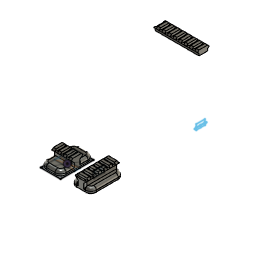
PhotoPicaTinny v1 (Autodesk Fusion 360 design; units mm, degrees)
Autodesk Fusion 360 part; units mm, degrees
sketch "Sketch1" plane through (0, 0, 0) normal (0, 0, 1) x (1, 0, 0)
  line L0 (18, 30) -> (-18, 30)
  line L1 (-18, 30) -> (-18, -30)
  line L2 (-18, -30) -> (18, -30)
  line L3 (18, -30) -> (18, 30)
  line L4 (18, 30) -> (-18, -30) construction
  line L5 (-18, 30) -> (18, -30) construction
  dimension "d1" = 36
  dimension "d2" = 60
  constraint horizontal L0
  constraint perpendicular L0 L1
  constraint parallel L0 L2
  constraint parallel L1 L3
  constraint coincident L4 origin
  constraint coincident L5 origin
  measures "d1" distance of L1.end L2.end
  measures "d2" distance of L0.end L1.end
extrude "Extrude1" add sketch "Sketch1" along normal blind 10 makes body 1
sketch "Sketch2" plane through (0, 0, 0) normal (0, 0, 1) x (1, 0, 0)
  line L0 (5, 30) -> (-5, 30)
  line L1 (-5, 30) -> (-5, -30)
  line L2 (-5, -30) -> (5, -30)
  line L3 (5, -30) -> (5, 30)
  line L4 (5, 30) -> (-5, -30) construction
  line L5 (-5, 30) -> (5, -30) construction
  line L6 (18, 30) -> (-18, 30)
  dimension "d5" = 10
  constraint horizontal L0
  constraint perpendicular L0 L1
  constraint parallel L0 L2
  constraint parallel L1 L3
  constraint coincident L4 origin
  constraint coincident L5 origin
  constraint coincident L0.start L6
  measures "d5" distance of L1.end L2.end
copy_body "CopyPasteBodies3" bodies 1 makes body 2
move_body "Move8" bodies 2 to x (1, 0, 0) y (0, 1, 0) z (0, 0, 1) at (0, 0, 0)
extrude "Extrude2" add sketch "Sketch2" along normal blind 13 bodies 1
sketch "Sketch3" plane through (0, 0, 0) normal (0, 0, 1) x (1, 0, 0)
sketch "Sketch4" plane through (0, 0, 0) normal (0, 0, 1) x (1, 0, 0)
  line L0 (18, 5) -> (-18, 5)
  line L1 (-18, 5) -> (-18, -5)
  line L2 (-18, -5) -> (18, -5)
  line L3 (18, -5) -> (18, 5)
  line L4 (18, 5) -> (-18, -5) construction
  line L5 (-18, 5) -> (18, -5) construction
  dimension "d8" = 10
  constraint horizontal L0
  constraint perpendicular L0 L1
  constraint parallel L0 L2
  constraint parallel L1 L3
  constraint coincident L4 origin
  constraint coincident L5 origin
  measures "d8" distance of L0.end L1.end
extrude "Extrude3" add sketch "Sketch1" along normal blind 10 separate body makes body 3
extrude "Extrude4" add sketch "Sketch4" along normal blind 12 separate body makes body 4
sketch "PicaMeasure2D" plane through (0, 0, 0) normal (1, 0, 0) x (0, 1, 0)
  line L0 (250.67, -64.32) -> (235, -64.32)
  line L1 (235, -64.32) -> (235, -55)
  line L2 (242.835, -61.32) -> (253.435, -61.32)
  line L3 (242.835, -61.32) -> (232.235, -61.32)
  line L4 (232.235, -61.32) -> (235, -64.32)
  line L5 (232.235, -61.32) -> (235, -58.7716)
  line L6 (249.8865, -60.32) -> (249.8865, -61.32)
  line L7 (242.835, -64.32) -> (242.835, -61.32)
  line L8 (242.835, -60.32) -> (249.8865, -60.32)
  line L9 (235, -55) -> (250.67, -55)
  line L10 (250.67, -55) -> (250.67, -64.32)
  line L11 (242.835, -61.32) -> (242.835, -60.32)
  line L12 (253.435, -61.32) -> (250.67, -58.7716)
  line L13 (242.835, -60.32) -> (235.7835, -60.32)
  line L14 (235.7835, -60.32) -> (235.7835, -61.32)
  line L15 (250.67, -64.32) -> (253.435, -61.32)
extrude "Extrude5" add sketch "PicaMeasure2D" along normal blind 5 separate body contours L2 L10 L12 | L1 L2 L3 L6 L8 L9 L10 L13 L14 | L1 L3 L5 makes body 5
extrude "Extrude6" add sketch "PicaMeasure2D" against normal blind 5 bodies 5
combine "Combine2" operation add target body 3 tool bodies 4
combine "Combine3" operation add target body 1 tool bodies 2
pattern_linear "R-Pattern1" count 8 spacing 10 along (1, 0, 0) of bodies 5 makes body 6 at (5, 240.2233, -60.6211) makes body 7 at (15, 240.2233, -60.6211) makes body 8 at (25, 240.2233, -60.6211) makes body 9 at (35, 240.2233, -60.6211) makes body 10 at (45, 240.2233, -60.6211) makes body 11 at (55, 240.2233, -60.6211) makes body 12 at (65, 240.2233, -60.6211)
combine "Combine1" operation add target body 5 tool bodies 6 7 8 9 10 11 12
move_body "Move1" bodies 5 to x (-1, 0, 0) y (0, 1, 0) z (0, 0, -1) at (0, 0, 0)
copy_body "CopyPasteBodies1" bodies 5 makes body 13
move_body "Move2" bodies 13 to x (1, 0, 0) y (0, 1, 0) z (0, 0, 1) at (57, -242.835, -43)
copy_body "CopyPasteBodies2" bodies 13 makes body 14
move_body "Move3" bodies 14 to x (0, 1, 0) y (-1, 0, 0) z (0, 0, 1) at (-25.835, 10.165, 0)
move_body "Move4" bodies 14 to x (1, 0, 0) y (0, 1, 0) z (0, 0, 1) at (25.835, -22.165, 1)
move_body "Move6" bodies 14 to x (1, 0, 0) y (0, 1, 0) z (0, 0, 1) at (0, -2, 0)
move_body "Move7" bodies 13 to x (1, 0, 0) y (0, 1, 0) z (0, 0, 1) at (-4, 0, 0)
sketch "Sketch6" plane through (58, 0, 0) normal (1, 0, 0) x (0, 1, 0)
  line L0 (-7.835, 21.32) -> (-10.6, 18.32)
  line L1 (-10.6, 18.32) -> (-7.835, 15.7716)
  line L2 (-7.835, 15.7716) -> (-7.835, 12)
  line L3 (-7.835, 12) -> (7.835, 12)
  line L4 (7.835, 12) -> (7.835, 15.7716)
  line L5 (7.835, 15.7716) -> (10.6, 18.32)
  line L6 (10.6, 18.32) -> (7.835, 21.32)
  line L7 (7.835, 21.32) -> (-7.835, 21.32)
  line L8 (8.4924, 22.82) -> (-8.4924, 22.82)
  line L9 (-8.4924, 22.82) -> (-12.7196, 18.2336)
  line L10 (-12.7196, 18.2336) -> (-9.335, 15.1142)
  line L11 (-9.335, 15.1142) -> (-9.335, 10.5)
  line L12 (-9.335, 10.5) -> (9.335, 10.5)
  line L13 (9.335, 10.5) -> (9.335, 15.1142)
  line L14 (9.335, 15.1142) -> (12.7196, 18.2336)
  line L15 (12.7196, 18.2336) -> (8.4924, 22.82)
  dimension "d48" = 1.5
extrude "Extrude8" add 1 faces at (-6, -5, 10.6667) along direction (0, -1, 0) blind 2.835 on bodies 3 bodies 3 13
extrude "Extrude10" cut sketch "Sketch1" along normal blind 30 keep common part bodies 3
extrude "Extrude11" add 1 faces at (-5, 10, 11) along direction (-1, 0, 0) blind 2.835 on bodies 1 bodies 1 14
extrude "Extrude12" add 1 faces at (5, -10, 11) along direction (1, 0, 0) blind 2.835 on bodies 1 bodies 1
extrude "Extrude13" cut sketch "Sketch1" along normal blind 25 keep common part bodies 1
move_body "Move5" bodies 1 to x (1, 0, 0) y (0, 1, 0) z (0, 0, 1) at (55, 0, 0)
extrude "Extrude15" add 1 faces at (6, 5, 10.6667) along direction (0, 1, 0) blind 2.835 on bodies 3 bodies 3
fillet "Fillet1" radius 10 8 edges at (37, -30, 5) (73, -30, 5) (73, 30, 5) (37, 30, 5) (18, -30, 5) (-18, -30, 5) (18, 30, 5) (-18, 30, 5) on bodies 1 3
fillet "Fillet2" radius 5 20 edges at (47.0825, 30, 10) (39.9289, 27.0711, 10) (37, 0, 10) (39.9289, -27.0711, 10) (47.0825, -30, 10) (62.9175, 30, 10) (70.0711, 27.0711, 10) (73, 0, 10) (70.0711, -27.0711, 10) (62.9175, -30, 10) (-18, -13.9175, 10) (-15.0711, -27.0711, 10) (0, -30, 10) (15.0711, -27.0711, 10) (18, -13.9175, 10) (18, 13.9175, 10) (15.0711, 27.0711, 10) (0, 30, 10) (-15.0711, 27.0711, 10) (-18, 13.9175, 10) on bodies 1 3
fillet "Fillet3" radius 2 16 edges at (70.0711, -27.0711, 0) (73, 0, 0) (70.0711, 27.0711, 0) (55, 30, 0) (39.9289, 27.0711, 0) (37, 0, 0) (39.9289, -27.0711, 0) (55, -30, 0) (15.0711, 27.0711, 0) (0, 30, 0) (-15.0711, 27.0711, 0) (-18, 0, 0) (-15.0711, -27.0711, 0) (0, -30, 0) (15.0711, -27.0711, 0) (18, 0, 0) on bodies 1 3
fillet "Fillet4" radius 3 8 edges at (47.165, -30, 10.8858) (62.835, -30, 10.8858) (47.165, 30, 10.8858) (62.835, 30, 10.8858) (-18, -7.835, 10.3858) (-18, 7.835, 10.3858) (18, -7.835, 10.3858) (18, 7.835, 10.3858) on bodies 1 3
named bodies: "PicaTinyVertical", "PicaTinyHorizontal", "PicaTinny"
